Autodesk Fusion 360 part; units mm, degrees
note: some values were not read from the file. Chosen so that the rebuilt part matches the saved one: which pieces of a blend or face edit are solid.
(part 2 of 2)
sketch "Sketch36" plane through (0, 20, 0) normal (0, 1, 0) x (-1, 0, 0)
  line L0 (-98, 0) -> (-112, 0)
  line L1 (-112, 0) -> (-112, -4.6)
  line L2 (-112, -4.6) -> (-98, -4.6)
  line L3 (-98, -4.6) -> (-98, 0)
  line L4 (-105, 0) -> (-105, -2.1)
  line L5 (-103, -2.8) -> (-107, -2.8)
  line L6 (-107, -2.8) -> (-107, -1.4)
  line L7 (-107, -1.4) -> (-103, -1.4)
  line L8 (-103, -1.4) -> (-103, -2.8)
  line L9 (-103, -2.8) -> (-107, -1.4) construction
  line L10 (-107, -2.8) -> (-103, -1.4) construction
  point P0 (-105, -2.1)
  dimension "d200" = 2.1
  dimension "d201" = 4
  dimension "d202" = 1.4
  constraint midpoint L0 L4.start
  constraint perpendicular L0 L4
  constraint horizontal L5
  constraint perpendicular L5 L6
  constraint parallel L5 L7
  constraint parallel L6 L8
  constraint coincident L9 P0
  constraint coincident L10 P0
  constraint coincident P0 L4.end
  measures "d200" distance of L4.start P0
  measures "d201" distance of L6.end L7.end
  measures "d202" distance of L5.end L6.end
extrude "Extrude37" cut sketch "Sketch36" against normal blind 1 contours L5 L6 L7 L8 bodies 1
sketch "Sketch37" plane through (0, 34, 0) normal (0, -1, 0) x (1, 0, 0)
  line L0 (112, 0) -> (98, 0)
  line L1 (98, 0) -> (98, -4.6)
  line L2 (98, -4.6) -> (112, -4.6)
  line L3 (112, -4.6) -> (112, 0)
  line L4 (105, 0) -> (105, -2.1)
  line L5 (107, -2.8) -> (103, -2.8)
  line L6 (103, -2.8) -> (103, -1.4)
  line L7 (103, -1.4) -> (107, -1.4)
  line L8 (107, -1.4) -> (107, -2.8)
  line L9 (107, -2.8) -> (103, -1.4) construction
  line L10 (103, -2.8) -> (107, -1.4) construction
  point P0 (105, -2.1)
  dimension "d205" = 2.1
  dimension "d206" = 4
  dimension "d207" = 1.4
  constraint midpoint L0 L4.start
  constraint perpendicular L0 L4
  constraint horizontal L5
  constraint perpendicular L5 L6
  constraint parallel L5 L7
  constraint parallel L6 L8
  constraint coincident L9 P0
  constraint coincident L10 P0
  constraint coincident P0 L4.end
  measures "d205" distance of L4.start P0
  measures "d206" distance of L6.end L7.end
  measures "d207" distance of L5.end L6.end
extrude "Extrude38" cut sketch "Sketch37" against normal blind 1 contours L5 L6 L7 L8 bodies 1
sketch "Sketch38" plane through (0, 50, 0) normal (0, -1, 0) x (1, 0, 0)
  line L0 (141, 0) -> (127, 0)
  line L1 (127, 0) -> (127, -4.6)
  line L2 (127, -4.6) -> (141, -4.6)
  line L3 (141, -4.6) -> (141, 0)
  line L4 (134, 0) -> (134, -2.1)
  line L5 (136, -2.8) -> (132, -2.8)
  line L6 (132, -2.8) -> (132, -1.4)
  line L7 (132, -1.4) -> (136, -1.4)
  line L8 (136, -1.4) -> (136, -2.8)
  line L9 (136, -2.8) -> (132, -1.4) construction
  line L10 (132, -2.8) -> (136, -1.4) construction
  point P0 (134, -2.1)
  dimension "d210" = 2.1
  dimension "d211" = 4
  dimension "d212" = 1.4
  constraint midpoint L0 L4.start
  constraint perpendicular L0 L4
  constraint horizontal L5
  constraint perpendicular L5 L6
  constraint parallel L5 L7
  constraint parallel L6 L8
  constraint coincident L9 P0
  constraint coincident L10 P0
  constraint coincident P0 L4.end
  measures "d210" distance of L4.start P0
  measures "d211" distance of L6.end L7.end
  measures "d212" distance of L5.end L6.end
extrude "Extrude39" cut sketch "Sketch38" against normal blind 1 contours L5 L6 L7 L8 bodies 1
sketch "Sketch39" plane through (0, 36, 0) normal (0, 1, 0) x (-1, 0, 0)
  line L0 (-127, 0) -> (-141, 0)
  line L1 (-141, 0) -> (-141, -4.6)
  line L2 (-141, -4.6) -> (-127, -4.6)
  line L3 (-127, -4.6) -> (-127, 0)
  line L4 (-134, 0) -> (-134, -2.1)
  line L5 (-132, -2.8) -> (-136, -2.8)
  line L6 (-136, -2.8) -> (-136, -1.4)
  line L7 (-136, -1.4) -> (-132, -1.4)
  line L8 (-132, -1.4) -> (-132, -2.8)
  line L9 (-132, -2.8) -> (-136, -1.4) construction
  line L10 (-136, -2.8) -> (-132, -1.4) construction
  point P0 (-134, -2.1)
  dimension "d215" = 2.1
  dimension "d216" = 4
  dimension "d217" = 1.4
  constraint midpoint L0 L4.start
  constraint perpendicular L0 L4
  constraint horizontal L5
  constraint perpendicular L5 L6
  constraint parallel L5 L7
  constraint parallel L6 L8
  constraint coincident L9 P0
  constraint coincident L10 P0
  constraint coincident P0 L4.end
  measures "d215" distance of L4.start P0
  measures "d216" distance of L6.end L7.end
  measures "d217" distance of L5.end L6.end
extrude "Extrude40" cut sketch "Sketch39" against normal blind 1 contours L5 L6 L7 L8 bodies 1
sketch "Sketch40" plane through (0, 17, 0) normal (0, 1, 0) x (-1, 0, 0)
  line L0 (-127, 0) -> (-141, 0)
  line L1 (-141, 0) -> (-141, -4.6)
  line L2 (-141, -4.6) -> (-127, -4.6)
  line L3 (-127, -4.6) -> (-127, 0)
  line L4 (-134, 0) -> (-134, -2.1)
  line L5 (-132, -2.8) -> (-136, -2.8)
  line L6 (-136, -2.8) -> (-136, -1.4)
  line L7 (-136, -1.4) -> (-132, -1.4)
  line L8 (-132, -1.4) -> (-132, -2.8)
  line L9 (-132, -2.8) -> (-136, -1.4) construction
  line L10 (-136, -2.8) -> (-132, -1.4) construction
  point P0 (-134, -2.1)
  dimension "d220" = 2.1
  dimension "d221" = 4
  dimension "d222" = 1.4
  constraint midpoint L0 L4.start
  constraint perpendicular L0 L4
  constraint horizontal L5
  constraint perpendicular L5 L6
  constraint parallel L5 L7
  constraint parallel L6 L8
  constraint coincident L9 P0
  constraint coincident L10 P0
  constraint coincident P0 L4.end
  measures "d220" distance of L4.start P0
  measures "d221" distance of L6.end L7.end
  measures "d222" distance of L5.end L6.end
extrude "Extrude41" cut sketch "Sketch40" against normal blind 1 contours L5 L6 L7 L8 bodies 1
sketch "Sketch41" plane through (0, 31, 0) normal (0, -1, 0) x (1, 0, 0)
  line L0 (141, 0) -> (127, 0)
  line L1 (127, 0) -> (127, -4.6)
  line L2 (127, -4.6) -> (141, -4.6)
  line L3 (141, -4.6) -> (141, 0)
  line L4 (134, 0) -> (134, -2.1)
  line L5 (136, -2.8) -> (132, -2.8)
  line L6 (132, -2.8) -> (132, -1.4)
  line L7 (132, -1.4) -> (136, -1.4)
  line L8 (136, -1.4) -> (136, -2.8)
  line L9 (136, -2.8) -> (132, -1.4) construction
  line L10 (132, -2.8) -> (136, -1.4) construction
  point P0 (134, -2.1)
  dimension "d225" = 2.1
  dimension "d226" = 4
  dimension "d227" = 1.4
  constraint midpoint L0 L4.start
  constraint perpendicular L0 L4
  constraint horizontal L5
  constraint perpendicular L5 L6
  constraint parallel L5 L7
  constraint parallel L6 L8
  constraint coincident L9 P0
  constraint coincident L10 P0
  constraint coincident P0 L4.end
  measures "d225" distance of L4.start P0
  measures "d226" distance of L6.end L7.end
  measures "d227" distance of L5.end L6.end
extrude "Extrude42" cut sketch "Sketch41" against normal blind 1 contours L5 L6 L7 L8 bodies 1
sketch "Sketch42" plane through (0, 34, 0) normal (0, -1, 0) x (1, 0, 0)
  line L0 (167, 0) -> (153, 0)
  line L1 (153, 0) -> (153, -4.6)
  line L2 (153, -4.6) -> (167, -4.6)
  line L3 (167, -4.6) -> (167, 0)
  line L4 (160, 0) -> (160, -2.1)
  line L5 (162, -2.8) -> (158, -2.8)
  line L6 (158, -2.8) -> (158, -1.4)
  line L7 (158, -1.4) -> (162, -1.4)
  line L8 (162, -1.4) -> (162, -2.8)
  line L9 (162, -2.8) -> (158, -1.4) construction
  line L10 (158, -2.8) -> (162, -1.4) construction
  point P0 (160, -2.1)
  dimension "d230" = 2.1
  dimension "d231" = 4
  dimension "d232" = 1.4
  constraint midpoint L0 L4.start
  constraint perpendicular L0 L4
  constraint horizontal L5
  constraint perpendicular L5 L6
  constraint parallel L5 L7
  constraint parallel L6 L8
  constraint coincident L9 P0
  constraint coincident L10 P0
  constraint coincident P0 L4.end
  measures "d230" distance of L4.start P0
  measures "d231" distance of L6.end L7.end
  measures "d232" distance of L5.end L6.end
extrude "Extrude43" cut sketch "Sketch42" against normal blind 1 contours L5 L6 L7 L8 bodies 1
sketch "Sketch43" plane through (0, 20, 0) normal (0, 1, 0) x (-1, 0, 0)
  line L0 (-153, 0) -> (-167, 0)
  line L1 (-167, 0) -> (-167, -4.6)
  line L2 (-167, -4.6) -> (-153, -4.6)
  line L3 (-153, -4.6) -> (-153, 0)
  line L4 (-160, 0) -> (-160, -2.1)
  line L5 (-158, -2.8) -> (-162, -2.8)
  line L6 (-162, -2.8) -> (-162, -1.4)
  line L7 (-162, -1.4) -> (-158, -1.4)
  line L8 (-158, -1.4) -> (-158, -2.8)
  line L9 (-158, -2.8) -> (-162, -1.4) construction
  line L10 (-162, -2.8) -> (-158, -1.4) construction
  point P0 (-160, -2.1)
  dimension "d235" = 2.1
  dimension "d236" = 4
  dimension "d237" = 1.4
  constraint midpoint L0 L4.start
  constraint perpendicular L0 L4
  constraint horizontal L5
  constraint perpendicular L5 L6
  constraint parallel L5 L7
  constraint parallel L6 L8
  constraint coincident L9 P0
  constraint coincident L10 P0
  constraint coincident P0 L4.end
  measures "d235" distance of L4.start P0
  measures "d236" distance of L6.end L7.end
  measures "d237" distance of L5.end L6.end
extrude "Extrude44" cut sketch "Sketch43" against normal blind 1 contours L5 L6 L7 L8 bodies 1
sketch "Sketch44" plane through (0, 1, 0) normal (0, 1, 0) x (-1, 0, 0)
  line L0 (-153, 0) -> (-167, 0)
  line L1 (-167, 0) -> (-167, -4.6)
  line L2 (-167, -4.6) -> (-153, -4.6)
  line L3 (-153, -4.6) -> (-153, 0)
  line L4 (-160, 0) -> (-160, -2.1)
  line L5 (-158, -2.8) -> (-162, -2.8)
  line L6 (-162, -2.8) -> (-162, -1.4)
  line L7 (-162, -1.4) -> (-158, -1.4)
  line L8 (-158, -1.4) -> (-158, -2.8)
  line L9 (-158, -2.8) -> (-162, -1.4) construction
  line L10 (-162, -2.8) -> (-158, -1.4) construction
  point P0 (-160, -2.1)
  dimension "d240" = 2.1
  dimension "d241" = 4
  dimension "d242" = 1.4
  constraint midpoint L0 L4.start
  constraint perpendicular L0 L4
  constraint horizontal L5
  constraint perpendicular L5 L6
  constraint parallel L5 L7
  constraint parallel L6 L8
  constraint coincident L9 P0
  constraint coincident L10 P0
  constraint coincident P0 L4.end
  measures "d240" distance of L4.start P0
  measures "d241" distance of L6.end L7.end
  measures "d242" distance of L5.end L6.end
extrude "Extrude45" cut sketch "Sketch44" against normal blind 1 contours L5 L6 L7 L8 bodies 1
sketch "Sketch45" plane through (0, 15, 0) normal (0, -1, 0) x (1, 0, 0)
  line L0 (167, 0) -> (153, 0)
  line L1 (153, 0) -> (153, -4.6)
  line L2 (153, -4.6) -> (167, -4.6)
  line L3 (167, -4.6) -> (167, 0)
  line L4 (160, 0) -> (160, -2.1)
  line L5 (162, -2.8) -> (158, -2.8)
  line L6 (158, -2.8) -> (158, -1.4)
  line L7 (158, -1.4) -> (162, -1.4)
  line L8 (162, -1.4) -> (162, -2.8)
  line L9 (162, -2.8) -> (158, -1.4) construction
  line L10 (158, -2.8) -> (162, -1.4) construction
  point P0 (160, -2.1)
  dimension "d245" = 2.1
  dimension "d246" = 4
  dimension "d247" = 1.4
  constraint midpoint L0 L4.start
  constraint perpendicular L0 L4
  constraint horizontal L5
  constraint perpendicular L5 L6
  constraint parallel L5 L7
  constraint parallel L6 L8
  constraint coincident L9 P0
  constraint coincident L10 P0
  constraint coincident P0 L4.end
  measures "d245" distance of L4.start P0
  measures "d246" distance of L6.end L7.end
  measures "d247" distance of L5.end L6.end
extrude "Extrude46" cut sketch "Sketch45" against normal blind 1 contours L5 L6 L7 L8 bodies 1
fillet "Fillet1" radius 1 8 edges at (-180.364, -66.364, 0) (-183, 0, 0) (-180.364, 66.364, 0) (0, 69, 0) (180.364, 66.364, 0) (183, 0, 0) (180.364, -66.364, 0) (0, -69, 0) on bodies 1
split "Split1" by plane through (0, 0, 0) normal (1, 0, 0) bodies 1 makes body 2 at (140.5828, -27.9, 0)
move_body "Move1" bodies 2 to x (1, 0, 0) y (0, 1, 0) z (0, 0, 1) at (10, 0, 0)
move_body "Move2" bodies 1 to x (1, 0, 0) y (0, 1, 0) z (0, 0, 1) at (-10, 0, 0)
sketch "Sketch46" plane through (0, 0, -4.6) normal (0, 0, -1) x (1, 0, 0)
  circle A0 centre (-65, -27) radius 12.5
  line L0 (-10, 27) -> (-10, 49)
  arc A1 (-20, 59) -> (-10, 49) centre (-10, 59) ccw
  line L1 (-20, 59) -> (-173, 59)
  arc A2 (-183, 49) -> (-173, 59) centre (-183, 59) ccw
  line L2 (-183, 49) -> (-183, -49)
  arc A3 (-173, -59) -> (-183, -49) centre (-183, -59) ccw
  line L3 (-173, -59) -> (-73, -59)
  arc A4 (-53, -59) -> (-73, -59) centre (-63, -59) ccw
  line L4 (-53, -59) -> (-22.344, -59)
  arc A5 (-21.3862, -60.2873) -> (-22.344, -59) centre (-22.344, -60) ccw
  line L5 (-21.3862, -60.2873) -> (-23.3586, -66.862)
  arc A6 (-26.2321, -69) -> (-23.3586, -66.862) centre (-26.2321, -66) ccw
  line L6 (-26.2321, -69) -> (-10, -69)
  line L7 (-10, -69) -> (-10, 13)
  line L8 (-10, 13) -> (-17, 13)
  line L9 (-17, 13) -> (-17, 27)
  line L10 (-17, 27) -> (-10, 27)
  line L11 (-163, -34) -> (-177, -34)
  line L12 (-177, -34) -> (-177, -20)
  line L13 (-177, -20) -> (-163, -20)
  line L14 (-163, -20) -> (-163, -34)
  line L15 (-89, 26) -> (-89, 40)
  line L16 (-89, 40) -> (-75, 40)
  line L17 (-75, 40) -> (-75, 26)
  line L18 (-75, 26) -> (-89, 26)
  line L19 (-108, -53) -> (-122, -53)
  line L20 (-122, -53) -> (-122, -39)
  line L21 (-122, -39) -> (-108, -39)
  line L22 (-108, -39) -> (-108, -53)
  line L23 (-96, -27) -> (-82, -27)
  line L24 (-82, -27) -> (-82, -41)
  line L25 (-82, -41) -> (-96, -41)
  line L26 (-96, -41) -> (-96, -27)
  line L27 (-137, -50) -> (-151, -50)
  line L28 (-151, -50) -> (-151, -36)
  line L29 (-151, -36) -> (-137, -36)
  line L30 (-137, -36) -> (-137, -50)
  line L31 (-70, 39) -> (-70, 53)
  line L32 (-70, 53) -> (-56, 53)
  line L33 (-56, 53) -> (-56, 39)
  line L34 (-56, 39) -> (-70, 39)
  circle A7 centre (-43, -54) radius 4
  circle A8 centre (-43, -20) radius 4
  circle A9 centre (-129.5, 0) radius 12.5
  line L35 (10, 3) -> (15, 3)
  line L36 (15, 3) -> (15, -49)
  line L37 (15, -49) -> (10, -49)
  line L38 (10, -49) -> (10, 3)
  line L39 (15, -49) -> (20, -49)
  line L40 (20, -49) -> (20, 3)
  line L41 (20, 3) -> (15, 3)
  line L42 (15, 3) -> (15, -49)
  line L43 (10, 44) -> (15, 44)
  line L44 (15, 44) -> (15, 32)
  line L45 (15, 32) -> (10, 32)
  line L46 (10, 32) -> (10, 44)
  line L47 (15, 44) -> (20, 44)
  line L48 (20, 44) -> (20, 32)
  line L49 (20, 32) -> (15, 32)
  line L50 (15, 32) -> (15, 44)
  line L51 (-10, 43.9) -> (-4.9, 43.9)
  line L52 (-10, 32.1) -> (-4.9, 32.1)
  line L53 (-10, 32.1) -> (-10, 43.9)
  line L54 (-4.9, 43.9) -> (-4.9, 32.1)
  line L55 (-4.9, 43.9) -> (-0.1, 43.9)
  line L56 (-0.1, 43.9) -> (-0.1, 32.1)
  line L57 (-0.1, 32.1) -> (-4.9, 32.1)
  line L58 (-10, -48.9) -> (-4.9, -48.9)
  line L59 (-10, 2.9) -> (-4.9, 2.9)
  line L60 (-4.9, 2.9) -> (-4.9, -48.9)
  line L61 (-10, -48.9) -> (-10, 2.9)
  line L62 (-4.9, 2.9) -> (-0.1, 2.9)
  line L63 (-4.9, -48.9) -> (-0.1, -48.9)
  line L64 (-0.1, -48.9) -> (-0.1, 2.9)
  dimension "d295" = 5.1
  dimension "d297" = 4.8
  dimension "d301" = 5.1
  dimension "d302" = 4.8
  constraint horizontal L35
  constraint vertical L36
  constraint horizontal L37
  constraint vertical L38
  constraint horizontal L39
  constraint vertical L40
  constraint horizontal L41
  constraint vertical L42
  constraint horizontal L43
  constraint vertical L44
  constraint horizontal L45
  constraint vertical L46
  constraint horizontal L47
  constraint vertical L48
  constraint horizontal L49
  constraint vertical L50
  constraint perpendicular L54 L55
  constraint perpendicular L55 L56
  constraint perpendicular L56 L57
  constraint perpendicular L7 L59
  constraint perpendicular L59 L61
  constraint perpendicular L60 L62
  constraint perpendicular L60 L63
  constraint perpendicular L62 L64
  measures "d295" distance of L51.start L51.end
  measures "d297" distance of L51.end L55.end
  measures "d301" distance of L59.start L59.end
  measures "d302" distance of L59.end L62.end
extrude "Extrude48" add sketch "Sketch46" against normal blind 4.6 separate body contours L54 L55 L56 L57 | L60 L62 L63 L64 makes body 3 at (-3.3, 14.3667, -4.6) makes body 4 at (-3.3, -36.0333, -4.6)
extrude "Extrude49" add sketch "Sketch46" against normal blind 2.2 contours L0 L51 L52 L53 L54 | L7 L58 L59 L60 L61 bodies 1 4 3
extrude "Extrude50" cut sketch "Sketch46" against normal blind 4.6 contours L36 L39 L40 L41 L42 | L44 L47 L48 L49 L50 bodies 2
extrude "Extrude51" cut sketch "Sketch46" against normal blind 2.4 contours L35 L36 L37 L38 L42 | L43 L44 L45 L46 L50 bodies 2
chamfer "Chamfer1" distance 0.4 angle 45 8 edges at (-180.5759, 58.0598, 0) (-180.5759, -59.9402, 0) (-65.4241, 59.9402, 0) (-12.6, -59, 0) (12.6, -59, 0) (60.5759, 59.9402, 0) (185.4241, -59.9402, 0) (185.4241, 58.0598, 0) on bodies 1 2
sketch "Sketch47" plane through (0, -69, 0) normal (0, -1, 0) x (1, 0, 0)
  line L0 (10, -1) -> (10, -16.6)
  line L1 (10, -16.6) -> (184, -16.6)
  line L2 (184, -16.6) -> (184, -1)
  line L3 (184, -1) -> (10, -1)
  line L4 (10, -8.8) -> (10, -3.8)
  line L5 (10, -3.8) -> (7.1132, -8.8)
  line L6 (10, -3.8) -> (15.7735, -3.8) construction
  line L7 (7.1132, -8.8) -> (10, -8.8)
  dimension "d305" = 5
  dimension "d306" = 120
  constraint midpoint L0 L4.start
  constraint parallel L0 L4
  constraint horizontal L6
  constraint perpendicular L4 L7
  measures "d305" distance of L4.start L4.end
  measures "d306" angle of L5 L6
extrude "Extrude52" add sketch "Sketch47" against normal blind 5 separate body contours L0 L4 L5 L7 makes body 5
move_body "Move4" bodies 5 to x (1, 0, 0) y (0, 1, 0) z (0, 0, 1) at (0, 1, 0)
copy_body "CopyPasteBodies1" bodies 5 makes body 6
move_body "Move5" bodies 6 to x (1, 0, 0) y (0, 1, 0) z (0, 0, 1) at (-20, 0, 0)
combine "Combine1" operation cut target body 1 tool bodies 6
move_face "OffsetFaces1" offset -0.1 4 faces at (-10.9623, -66.3333, -5.4667) (-10.9623, -63, -7.1333) (-11.9245, -64.6667, -8.8) (-10.9623, -68, -7.1333) on bodies 1
sketch "Sketch48" plane through (0, 0, 0) normal (0, 0, 1) x (-1, 0, 0)
  arc A0 (10, 56) -> (10, 62) centre (10, 59) ccw
  line L0 (10, 56) -> (10, 27)
  line L1 (10, 27) -> (17, 27)
  line L2 (17, 27) -> (17, 13)
  line L3 (17, 13) -> (10, 13)
  line L4 (10, 13) -> (10, -68)
  line L5 (10, -68) -> (184, -68)
  arc A1 (184, -68) -> (192, -60) centre (184, -60) ccw
  line L6 (192, -60) -> (192, 60)
  arc A2 (192, 60) -> (184, 68) centre (184, 60) ccw
  line L7 (184, 68) -> (10, 68)
  line L8 (10, 68) -> (10, 62)
  circle A3 centre (183, 59) radius 3
  circle A4 centre (43, -54) radius 3.5
  circle A5 centre (43, -20) radius 3.5
  line L9 (70, 53) -> (70, 39)
  line L10 (70, 39) -> (56, 39)
  line L11 (56, 39) -> (56, 53)
  line L12 (56, 53) -> (70, 53)
  line L13 (151, -50) -> (137, -50)
  line L14 (137, -50) -> (137, -36)
  line L15 (137, -36) -> (151, -36)
  line L16 (151, -36) -> (151, -50)
  line L17 (82, -27) -> (96, -27)
  line L18 (96, -27) -> (96, -41)
  line L19 (96, -41) -> (82, -41)
  line L20 (82, -41) -> (82, -27)
  line L21 (122, -53) -> (108, -53)
  line L22 (108, -53) -> (108, -39)
  line L23 (108, -39) -> (122, -39)
  line L24 (122, -39) -> (122, -53)
  line L25 (89, 40) -> (89, 26)
  line L26 (89, 26) -> (75, 26)
  line L27 (75, 26) -> (75, 40)
  line L28 (75, 40) -> (89, 40)
  line L29 (177, -34) -> (163, -34)
  line L30 (163, -34) -> (163, -20)
  line L31 (163, -20) -> (177, -20)
  line L32 (177, -20) -> (177, -34)
  circle A6 centre (183, -59) radius 3
  circle A7 centre (63, -59) radius 3
  line L33 (22, 13) -> (36, 13)
  line L34 (36, 13) -> (36, 27)
  line L35 (36, 27) -> (22, 27)
  line L36 (22, 27) -> (22, 13)
  line L37 (-22, 13) -> (-36, 13)
  line L38 (-36, 13) -> (-36, 27)
  line L39 (-36, 27) -> (-22, 27)
  line L40 (-22, 27) -> (-22, 13)
  dimension "d310" = 14
  dimension "d311" = 14
  dimension "d312" = 14
  dimension "d313" = 14
  constraint horizontal L33
  constraint vertical L34
  constraint horizontal L35
  constraint vertical L36
  constraint horizontal L37
  constraint vertical L38
  constraint horizontal L39
  constraint vertical L40
  measures "d310" distance of L33.start L33.end
  measures "d311" distance of L33.start L35.end
  measures "d312" distance of L37.start L37.end
  measures "d313" distance of L37.start L39.end
extrude "Extrude53" cut sketch "Sketch48" against normal blind 4.6 contours L33 L34 L35 L36 | L37 L38 L39 L40 bodies 1 2
sketch "Sketch49" plane through (0, -27, 0) normal (0, 1, 0) x (-1, 0, 0)
  line L0 (-22, 0) -> (-36, 0)
  line L1 (-36, 0) -> (-36, -4.6)
  line L2 (-36, -4.6) -> (-22, -4.6)
  line L3 (-22, -4.6) -> (-22, 0)
  line L4 (-29, 0) -> (-29, -2.1)
  line L5 (-27, -2.8) -> (-31, -2.8)
  line L6 (-31, -2.8) -> (-31, -1.4)
  line L7 (-31, -1.4) -> (-27, -1.4)
  line L8 (-27, -1.4) -> (-27, -2.8)
  line L9 (-27, -2.8) -> (-31, -1.4) construction
  line L10 (-31, -2.8) -> (-27, -1.4) construction
  line L11 (29, 0) -> (29, -2.1)
  line L12 (31, -2.8) -> (27, -2.8)
  line L13 (27, -2.8) -> (27, -1.4)
  line L14 (27, -1.4) -> (31, -1.4)
  line L15 (31, -1.4) -> (31, -2.8)
  line L16 (31, -2.8) -> (27, -1.4) construction
  line L17 (27, -2.8) -> (31, -1.4) construction
  point P0 (-29, -2.1)
  point P1 (29, -2.1)
  dimension "d316" = 2.1
  dimension "d317" = 4
  dimension "d318" = 1.4
  dimension "d319" = 2.1
  dimension "d320" = 4
  dimension "d321" = 1.4
  constraint midpoint L0 L4.start
  constraint perpendicular L0 L4
  constraint horizontal L5
  constraint perpendicular L5 L6
  constraint parallel L5 L7
  constraint parallel L6 L8
  constraint coincident L9 P0
  constraint coincident L10 P0
  constraint coincident P0 L4.end
  constraint vertical L11
  constraint horizontal L12
  constraint perpendicular L12 L13
  constraint parallel L12 L14
  constraint parallel L13 L15
  constraint coincident L16 P1
  constraint coincident L17 P1
  constraint coincident P1 L11.end
  measures "d316" distance of L4.start P0
  measures "d317" distance of L6.end L7.end
  measures "d318" distance of L5.end L6.end
  measures "d319" distance of L11.start P1
  measures "d320" distance of L13.end L14.end
  measures "d321" distance of L12.end L13.end
sketch "Sketch50" plane through (0, -13, 0) normal (0, -1, 0) x (1, 0, 0)
  line L0 (-22, 0) -> (-36, 0)
  line L1 (-36, 0) -> (-36, -4.6)
  line L2 (-36, -4.6) -> (-22, -4.6)
  line L3 (-22, -4.6) -> (-22, 0)
  line L4 (-29, 0) -> (-29, -2.1)
  line L5 (-27, -2.8) -> (-31, -2.8)
  line L6 (-31, -2.8) -> (-31, -1.4)
  line L7 (-31, -1.4) -> (-27, -1.4)
  line L8 (-27, -1.4) -> (-27, -2.8)
  line L9 (-27, -2.8) -> (-31, -1.4) construction
  line L10 (-31, -2.8) -> (-27, -1.4) construction
  line L11 (29, 0) -> (29, -2.1)
  line L12 (31, -2.8) -> (27, -2.8)
  line L13 (27, -2.8) -> (27, -1.4)
  line L14 (27, -1.4) -> (31, -1.4)
  line L15 (31, -1.4) -> (31, -2.8)
  line L16 (31, -2.8) -> (27, -1.4) construction
  line L17 (27, -2.8) -> (31, -1.4) construction
  point P0 (-29, -2.1)
  point P1 (29, -2.1)
  dimension "d322" = 2.1
  dimension "d323" = 4
  dimension "d324" = 1.4
  dimension "d325" = 2.1
  dimension "d326" = 4
  dimension "d327" = 1.4
  constraint midpoint L0 L4.start
  constraint perpendicular L0 L4
  constraint horizontal L5
  constraint perpendicular L5 L6
  constraint parallel L5 L7
  constraint parallel L6 L8
  constraint coincident L9 P0
  constraint coincident L10 P0
  constraint coincident P0 L4.end
  constraint vertical L11
  constraint horizontal L12
  constraint perpendicular L12 L13
  constraint parallel L12 L14
  constraint parallel L13 L15
  constraint coincident L16 P1
  constraint coincident L17 P1
  constraint coincident P1 L11.end
  measures "d322" distance of L4.start P0
  measures "d323" distance of L6.end L7.end
  measures "d324" distance of L5.end L6.end
  measures "d325" distance of L11.start P1
  measures "d326" distance of L13.end L14.end
  measures "d327" distance of L12.end L13.end
extrude "Extrude54" cut sketch "Sketch50" against normal blind 1 contours L5 L6 L7 L8 | L12 L13 L14 L15 bodies 1 2
extrude "Extrude55" cut sketch "Sketch49" against normal blind 1 contours L5 L6 L7 L8 | L12 L13 L14 L15 bodies 1 2
hidden bodies 1
